Autodesk Fusion 360 part; units mm, degrees
note: some values were not read from the file. Set by a fixed rule: which sketch regions a step uses.
(part 3 of 3)
  arc A262 (-92.225, 45.1) -> (-92.725, 44.6) centre (-92.225, 44.6) ccw
  line L262 (-92.225, 45.1) -> (-79.225, 45.1)
  arc A263 (-78.725, 44.6) -> (-79.225, 45.1) centre (-79.225, 44.6) ccw
  line L263 (-78.725, 44.6) -> (-78.725, 31.6)
  arc A264 (-112.5625, 69.2) -> (-112.0625, 69.7) centre (-112.5625, 69.7) ccw
  line L264 (-112.5625, 69.2) -> (-125.5625, 69.2)
  arc A265 (-126.0625, 69.7) -> (-125.5625, 69.2) centre (-125.5625, 69.7) ccw
  line L265 (-126.0625, 69.7) -> (-126.0625, 82.7)
  arc A266 (-125.5625, 83.2) -> (-126.0625, 82.7) centre (-125.5625, 82.7) ccw
  line L266 (-125.5625, 83.2) -> (-112.5625, 83.2)
  arc A267 (-112.0625, 82.7) -> (-112.5625, 83.2) centre (-112.5625, 82.7) ccw
  line L267 (-112.0625, 82.7) -> (-112.0625, 69.7)
  arc A268 (-177.9688, 108.3) -> (-177.4687, 108.8) centre (-177.9688, 108.8) ccw
  line L268 (-177.9688, 108.3) -> (-183.9688, 108.3)
  arc A269 (-184.4688, 108.8) -> (-183.9688, 108.3) centre (-183.9688, 108.8) ccw
  line L269 (-184.4688, 108.8) -> (-184.4688, 122.8)
  arc A270 (-183.9688, 123.3) -> (-184.4687, 122.8) centre (-183.9687, 122.8) ccw
  line L270 (-183.9688, 123.3) -> (-177.9688, 123.3)
  arc A271 (-177.4688, 122.8) -> (-177.9688, 123.3) centre (-177.9688, 122.8) ccw
  line L271 (-177.4688, 122.8) -> (-177.4687, 108.8)
  arc A272 (-331.6375, 2.525) -> (-331.1375, 3.025) centre (-331.6375, 3.025) ccw
  line L272 (-331.6375, 2.525) -> (-344.6375, 2.525)
  arc A273 (-345.1375, 3.025) -> (-344.6375, 2.525) centre (-344.6375, 3.025) ccw
  line L273 (-345.1375, 3.025) -> (-345.1375, 16.025)
  arc A274 (-344.6375, 16.525) -> (-345.1375, 16.025) centre (-344.6375, 16.025) ccw
  line L274 (-344.6375, 16.525) -> (-331.6375, 16.525)
  arc A275 (-331.1375, 16.025) -> (-331.6375, 16.525) centre (-331.6375, 16.025) ccw
  line L275 (-331.1375, 16.025) -> (-331.1375, 3.025)
  arc A276 (-83.9875, 88.25) -> (-83.4875, 88.75) centre (-83.9875, 88.75) ccw
  line L276 (-83.9875, 88.25) -> (-96.9875, 88.25)
  arc A277 (-97.4875, 88.75) -> (-96.9875, 88.25) centre (-96.9875, 88.75) ccw
  line L277 (-97.4875, 88.75) -> (-97.4875, 101.75)
  arc A278 (-96.9875, 102.25) -> (-97.4875, 101.75) centre (-96.9875, 101.75) ccw
  line L278 (-96.9875, 102.25) -> (-83.9875, 102.25)
  arc A279 (-83.4875, 101.75) -> (-83.9875, 102.25) centre (-83.9875, 101.75) ccw
  line L279 (-83.4875, 101.75) -> (-83.4875, 88.75)
  arc A280 (-5.4063, 88.25) -> (-4.9063, 88.75) centre (-5.4062, 88.75) ccw
  line L280 (-5.4062, 88.25) -> (-18.4063, 88.25)
  arc A281 (-18.9062, 88.75) -> (-18.4063, 88.25) centre (-18.4062, 88.75) ccw
  line L281 (-18.9062, 88.75) -> (-18.9063, 101.75)
  arc A282 (-18.4062, 102.25) -> (-18.9063, 101.75) centre (-18.4063, 101.75) ccw
  line L282 (-18.4062, 102.25) -> (-5.4063, 102.25)
  arc A283 (-4.9062, 101.75) -> (-5.4063, 102.25) centre (-5.4062, 101.75) ccw
  line L283 (-4.9062, 101.75) -> (-4.9063, 88.75)
  arc A284 (-5.4063, 107.3) -> (-4.9062, 107.8) centre (-5.4063, 107.8) ccw
  line L284 (-5.4062, 107.3) -> (-18.4063, 107.3)
  arc A285 (-18.9062, 107.8) -> (-18.4063, 107.3) centre (-18.4062, 107.8) ccw
  line L285 (-18.9062, 107.8) -> (-18.9063, 120.8)
  arc A286 (-18.4062, 121.3) -> (-18.9063, 120.8) centre (-18.4062, 120.8) ccw
  line L286 (-18.4062, 121.3) -> (-5.4063, 121.3)
  arc A287 (-4.9062, 120.8) -> (-5.4063, 121.3) centre (-5.4063, 120.8) ccw
  line L287 (-4.9062, 120.8) -> (-4.9062, 107.8)
  arc A288 (-243.5313, 107.3) -> (-243.0313, 107.8) centre (-243.5312, 107.8) ccw
  line L288 (-243.5313, 107.3) -> (-256.5313, 107.3)
  arc A289 (-257.0312, 107.8) -> (-256.5312, 107.3) centre (-256.5312, 107.8) ccw
  line L289 (-257.0312, 107.8) -> (-257.0313, 120.8)
  arc A290 (-256.5312, 121.3) -> (-257.0312, 120.8) centre (-256.5312, 120.8) ccw
  line L290 (-256.5312, 121.3) -> (-243.5312, 121.3)
  arc A291 (-243.0313, 120.8) -> (-243.5313, 121.3) centre (-243.5313, 120.8) ccw
  line L291 (-243.0312, 120.8) -> (-243.0312, 107.8)
  arc A292 (-244.6183, 89.25) -> (-244.1182, 89.75) centre (-244.6183, 89.75) ccw
  line L292 (-244.6183, 89.25) -> (-250.6182, 89.25)
  arc A293 (-251.1182, 89.75) -> (-250.6182, 89.25) centre (-250.6182, 89.75) ccw
  line L293 (-251.1182, 89.75) -> (-251.1182, 103.75)
  arc A294 (-250.6182, 104.25) -> (-251.1182, 103.75) centre (-250.6182, 103.75) ccw
  line L294 (-250.6182, 104.25) -> (-244.6183, 104.25)
  arc A295 (-244.1183, 103.75) -> (-244.6183, 104.25) centre (-244.6182, 103.75) ccw
  line L295 (-244.1182, 103.75) -> (-244.1182, 89.75)
  arc A296 (-88.75, 50.15) -> (-88.25, 50.65) centre (-88.75, 50.65) ccw
  line L296 (-88.75, 50.15) -> (-101.75, 50.15)
  arc A297 (-102.25, 50.65) -> (-101.75, 50.15) centre (-101.75, 50.65) ccw
  line L297 (-102.25, 50.65) -> (-102.25, 63.65)
  arc A298 (-101.75, 64.15) -> (-102.25, 63.65) centre (-101.75, 63.65) ccw
  line L298 (-101.75, 64.15) -> (-88.75, 64.15)
  arc A299 (-88.25, 63.65) -> (-88.75, 64.15) centre (-88.75, 63.65) ccw
  line L299 (-88.25, 63.65) -> (-88.25, 50.65)
  arc A300 (-293.5375, 2.525) -> (-293.0375, 3.025) centre (-293.5375, 3.025) ccw
  line L300 (-293.5375, 2.525) -> (-306.5375, 2.525)
  arc A301 (-307.0375, 3.025) -> (-306.5375, 2.525) centre (-306.5375, 3.025) ccw
  line L301 (-307.0375, 3.025) -> (-307.0375, 16.025)
  arc A302 (-306.5375, 16.525) -> (-307.0375, 16.025) centre (-306.5375, 16.025) ccw
  line L302 (-306.5375, 16.525) -> (-293.5375, 16.525)
  arc A303 (-293.0375, 16.025) -> (-293.5375, 16.525) centre (-293.5375, 16.025) ccw
  line L303 (-293.0375, 16.025) -> (-293.0375, 3.025)
  arc A304 (-293.5375, 50.15) -> (-293.0375, 50.65) centre (-293.5375, 50.65) ccw
  line L304 (-293.5375, 50.15) -> (-306.5375, 50.15)
  arc A305 (-307.0375, 50.65) -> (-306.5375, 50.15) centre (-306.5375, 50.65) ccw
  line L305 (-307.0375, 50.65) -> (-307.0375, 63.65)
  arc A306 (-306.5375, 64.15) -> (-307.0375, 63.65) centre (-306.5375, 63.65) ccw
  line L306 (-306.5375, 64.15) -> (-293.5375, 64.15)
  arc A307 (-293.0375, 63.65) -> (-293.5375, 64.15) centre (-293.5375, 63.65) ccw
  line L307 (-293.0375, 63.65) -> (-293.0375, 50.65)
  arc A308 (-69.7, 50.15) -> (-69.2, 50.65) centre (-69.7, 50.65) ccw
  line L308 (-69.7, 50.15) -> (-82.7, 50.15)
  arc A309 (-83.2, 50.65) -> (-82.7, 50.15) centre (-82.7, 50.65) ccw
  line L309 (-83.2, 50.65) -> (-83.2, 63.65)
  arc A310 (-82.7, 64.15) -> (-83.2, 63.65) centre (-82.7, 63.65) ccw
  line L310 (-82.7, 64.15) -> (-69.7, 64.15)
  arc A311 (-69.2, 63.65) -> (-69.7, 64.15) centre (-69.7, 63.65) ccw
  line L311 (-69.2, 63.65) -> (-69.2, 50.65)
  arc A312 (-3.025, 31.1) -> (-2.525, 31.6) centre (-3.025, 31.6) ccw
  line L312 (-3.025, 31.1) -> (-16.025, 31.1)
  arc A313 (-16.525, 31.6) -> (-16.025, 31.1) centre (-16.025, 31.6) ccw
  line L313 (-16.525, 31.6) -> (-16.525, 44.6)
  arc A314 (-16.025, 45.1) -> (-16.525, 44.6) centre (-16.025, 44.6) ccw
  line L314 (-16.025, 45.1) -> (-3.025, 45.1)
  arc A315 (-2.525, 44.6) -> (-3.025, 45.1) centre (-3.025, 44.6) ccw
  line L315 (-2.525, 44.6) -> (-2.525, 31.6)
  arc A316 (-331.6375, 107.3) -> (-331.1375, 107.8) centre (-331.6375, 107.8) ccw
  line L316 (-331.6375, 107.3) -> (-344.6375, 107.3)
  arc A317 (-345.1375, 107.8) -> (-344.6375, 107.3) centre (-344.6375, 107.8) ccw
  line L317 (-345.1375, 107.8) -> (-345.1375, 120.8)
  arc A318 (-344.6375, 121.3) -> (-345.1375, 120.8) centre (-344.6375, 120.8) ccw
  line L318 (-344.6375, 121.3) -> (-331.6375, 121.3)
  arc A319 (-331.1375, 120.8) -> (-331.6375, 121.3) centre (-331.6375, 120.8) ccw
  line L319 (-331.1375, 120.8) -> (-331.1375, 107.8)
  arc A320 (-155.425, 31.1) -> (-154.925, 31.6) centre (-155.425, 31.6) ccw
  line L320 (-155.425, 31.1) -> (-168.425, 31.1)
  arc A321 (-168.925, 31.6) -> (-168.425, 31.1) centre (-168.425, 31.6) ccw
  line L321 (-168.925, 31.6) -> (-168.925, 44.6)
  arc A322 (-168.425, 45.1) -> (-168.925, 44.6) centre (-168.425, 44.6) ccw
  line L322 (-168.425, 45.1) -> (-155.425, 45.1)
  arc A323 (-154.925, 44.6) -> (-155.425, 45.1) centre (-155.425, 44.6) ccw
  line L323 (-154.925, 44.6) -> (-154.925, 31.6)
  arc A324 (-77.9688, 108.3) -> (-77.4687, 108.8) centre (-77.9688, 108.8) ccw
  line L324 (-77.9688, 108.3) -> (-83.9688, 108.3)
  arc A325 (-84.4688, 108.8) -> (-83.9688, 108.3) centre (-83.9687, 108.8) ccw
  line L325 (-84.4688, 108.8) -> (-84.4687, 122.8)
  arc A326 (-83.9688, 123.3) -> (-84.4687, 122.8) centre (-83.9688, 122.8) ccw
  line L326 (-83.9688, 123.3) -> (-77.9688, 123.3)
  arc A327 (-77.4688, 122.8) -> (-77.9688, 123.3) centre (-77.9688, 122.8) ccw
  line L327 (-77.4688, 122.8) -> (-77.4687, 108.8)
  arc A328 (-275.638, 32.1) -> (-275.138, 32.6) centre (-275.638, 32.6) ccw
  line L328 (-275.638, 32.1) -> (-281.638, 32.1)
  arc A329 (-282.138, 32.6) -> (-281.638, 32.1) centre (-281.638, 32.6) ccw
  line L329 (-282.138, 32.6) -> (-282.138, 46.6)
  arc A330 (-281.638, 47.1) -> (-282.138, 46.6) centre (-281.638, 46.6) ccw
  line L330 (-281.638, 47.1) -> (-275.638, 47.1)
  arc A331 (-275.138, 46.6) -> (-275.638, 47.1) centre (-275.638, 46.6) ccw
  line L331 (-275.138, 46.6) -> (-275.138, 32.6)
  arc A332 (-145.9, 50.15) -> (-145.4, 50.65) centre (-145.9, 50.65) ccw
  line L332 (-145.9, 50.15) -> (-158.9, 50.15)
  arc A333 (-159.4, 50.65) -> (-158.9, 50.15) centre (-158.9, 50.65) ccw
  line L333 (-159.4, 50.65) -> (-159.4, 63.65)
  arc A334 (-158.9, 64.15) -> (-159.4, 63.65) centre (-158.9, 63.65) ccw
  line L334 (-158.9, 64.15) -> (-145.9, 64.15)
  arc A335 (-145.4, 63.65) -> (-145.9, 64.15) centre (-145.9, 63.65) ccw
  line L335 (-145.4, 63.65) -> (-145.4, 50.65)
  arc A336 (-198.2875, 88.25) -> (-197.7875, 88.75) centre (-198.2875, 88.75) ccw
  line L336 (-198.2875, 88.25) -> (-211.2875, 88.25)
  arc A337 (-211.7875, 88.75) -> (-211.2875, 88.25) centre (-211.2875, 88.75) ccw
  line L337 (-211.7875, 88.75) -> (-211.7875, 101.75)
  arc A338 (-211.2875, 102.25) -> (-211.7875, 101.75) centre (-211.2875, 101.75) ccw
  line L338 (-211.2875, 102.25) -> (-198.2875, 102.25)
  arc A339 (-197.7875, 101.75) -> (-198.2875, 102.25) centre (-198.2875, 101.75) ccw
  line L339 (-197.7875, 101.75) -> (-197.7875, 88.75)
  arc A340 (-195.9063, 107.3) -> (-195.4063, 107.8) centre (-195.9063, 107.8) ccw
  line L340 (-195.9063, 107.3) -> (-208.9062, 107.3)
  arc A341 (-209.4062, 107.8) -> (-208.9062, 107.3) centre (-208.9062, 107.8) ccw
  line L341 (-209.4062, 107.8) -> (-209.4062, 120.8)
  arc A342 (-208.9062, 121.3) -> (-209.4063, 120.8) centre (-208.9062, 120.8) ccw
  line L342 (-208.9062, 121.3) -> (-195.9063, 121.3)
  arc A343 (-195.4063, 120.8) -> (-195.9063, 121.3) centre (-195.9063, 120.8) ccw
  line L343 (-195.4063, 120.8) -> (-195.4063, 107.8)
  arc A344 (-64.9375, 88.25) -> (-64.4375, 88.75) centre (-64.9375, 88.75) ccw
  line L344 (-64.9375, 88.25) -> (-77.9375, 88.25)
  arc A345 (-78.4375, 88.75) -> (-77.9375, 88.25) centre (-77.9375, 88.75) ccw
  line L345 (-78.4375, 88.75) -> (-78.4375, 101.75)
  arc A346 (-77.9375, 102.25) -> (-78.4375, 101.75) centre (-77.9375, 101.75) ccw
  line L346 (-77.9375, 102.25) -> (-64.9375, 102.25)
  arc A347 (-64.4375, 101.75) -> (-64.9375, 102.25) centre (-64.9375, 101.75) ccw
  line L347 (-64.4375, 101.75) -> (-64.4375, 88.75)
  arc A348 (-60.175, 2.525) -> (-59.675, 3.025) centre (-60.175, 3.025) ccw
  line L348 (-60.175, 2.525) -> (-73.175, 2.525)
  arc A349 (-73.675, 3.025) -> (-73.175, 2.525) centre (-73.175, 3.025) ccw
  line L349 (-73.675, 3.025) -> (-73.675, 16.025)
  arc A350 (-73.175, 16.525) -> (-73.675, 16.025) centre (-73.175, 16.025) ccw
  line L350 (-73.175, 16.525) -> (-60.175, 16.525)
  arc A351 (-59.675, 16.025) -> (-60.175, 16.525) centre (-60.175, 16.025) ccw
  line L351 (-59.675, 16.025) -> (-59.675, 3.025)
  arc A352 (-331.6375, 31.1) -> (-331.1375, 31.6) centre (-331.6375, 31.6) ccw
  line L352 (-331.6375, 31.1) -> (-344.6375, 31.1)
  arc A353 (-345.1375, 31.6) -> (-344.6375, 31.1) centre (-344.6375, 31.6) ccw
  line L353 (-345.1375, 31.6) -> (-345.1375, 44.6)
  arc A354 (-344.6375, 45.1) -> (-345.1375, 44.6) centre (-344.6375, 44.6) ccw
  line L354 (-344.6375, 45.1) -> (-331.6375, 45.1)
  arc A355 (-331.1375, 44.6) -> (-331.6375, 45.1) centre (-331.6375, 44.6) ccw
  line L355 (-331.1375, 44.6) -> (-331.1375, 31.6)
  arc A356 (-280.8438, 60.175) -> (-280.3438, 59.675) centre (-280.3438, 60.175) ccw
  line L356 (-280.8438, 60.175) -> (-280.8438, 73.175)
  arc A357 (-280.3438, 73.675) -> (-280.8438, 73.175) centre (-280.3438, 73.175) ccw
  line L357 (-280.3438, 73.675) -> (-267.3438, 73.675)
  arc A358 (-266.8438, 73.175) -> (-267.3438, 73.675) centre (-267.3438, 73.175) ccw
  line L358 (-266.8438, 73.175) -> (-266.8437, 60.175)
  arc A359 (-267.3438, 59.675) -> (-266.8438, 60.175) centre (-267.3438, 60.175) ccw
  line L359 (-267.3438, 59.675) -> (-280.3438, 59.675)
  arc A360 (-126.85, 2.525) -> (-126.35, 3.025) centre (-126.85, 3.025) ccw
  line L360 (-126.85, 2.525) -> (-139.85, 2.525)
  arc A361 (-140.35, 3.025) -> (-139.85, 2.525) centre (-139.85, 3.025) ccw
  line L361 (-140.35, 3.025) -> (-140.35, 16.025)
  arc A362 (-139.85, 16.525) -> (-140.35, 16.025) centre (-139.85, 16.025) ccw
  line L362 (-139.85, 16.525) -> (-126.85, 16.525)
  arc A363 (-126.35, 16.025) -> (-126.85, 16.525) centre (-126.85, 16.025) ccw
  line L363 (-126.35, 16.025) -> (-126.35, 3.025)
  arc A364 (-53.0313, 107.3) -> (-52.5312, 107.8) centre (-53.0313, 107.8) ccw
  line L364 (-53.0313, 107.3) -> (-66.0312, 107.3)
  arc A365 (-66.5312, 107.8) -> (-66.0312, 107.3) centre (-66.0312, 107.8) ccw
  line L365 (-66.5312, 107.8) -> (-66.5313, 120.8)
  arc A366 (-66.0313, 121.3) -> (-66.5313, 120.8) centre (-66.0312, 120.8) ccw
  line L366 (-66.0312, 121.3) -> (-53.0312, 121.3)
  arc A367 (-52.5313, 120.8) -> (-53.0313, 121.3) centre (-53.0312, 120.8) ccw
  line L367 (-52.5313, 120.8) -> (-52.5312, 107.8)
  arc A368 (-184, 50.15) -> (-183.5, 50.65) centre (-184, 50.65) ccw
  line L368 (-184, 50.15) -> (-197, 50.15)
  arc A369 (-197.5, 50.65) -> (-197, 50.15) centre (-197, 50.65) ccw
  line L369 (-197.5, 50.65) -> (-197.5, 63.65)
  arc A370 (-197, 64.15) -> (-197.5, 63.65) centre (-197, 63.65) ccw
  line L370 (-197, 64.15) -> (-184, 64.15)
  arc A371 (-183.5, 63.65) -> (-184, 64.15) centre (-184, 63.65) ccw
  line L371 (-183.5, 63.65) -> (-183.5, 50.65)
  arc A372 (-269.725, 2.525) -> (-269.225, 3.025) centre (-269.725, 3.025) ccw
  line L372 (-269.725, 2.525) -> (-282.725, 2.525)
  arc A373 (-283.225, 3.025) -> (-282.725, 2.525) centre (-282.725, 3.025) ccw
  line L373 (-283.225, 3.025) -> (-283.225, 16.025)
  arc A374 (-282.725, 16.525) -> (-283.225, 16.025) centre (-282.725, 16.025) ccw
  line L374 (-282.725, 16.525) -> (-269.725, 16.525)
  arc A375 (-269.225, 16.025) -> (-269.725, 16.525) centre (-269.725, 16.025) ccw
  line L375 (-269.225, 16.025) -> (-269.225, 3.025)
  arc A376 (-126.85, 50.15) -> (-126.35, 50.65) centre (-126.85, 50.65) ccw
  line L376 (-126.85, 50.15) -> (-139.85, 50.15)
  arc A377 (-140.35, 50.65) -> (-139.85, 50.15) centre (-139.85, 50.65) ccw
  line L377 (-140.35, 50.65) -> (-140.35, 63.65)
  arc A378 (-139.85, 64.15) -> (-140.35, 63.65) centre (-139.85, 63.65) ccw
  line L378 (-139.85, 64.15) -> (-126.85, 64.15)
  arc A379 (-126.35, 63.65) -> (-126.85, 64.15) centre (-126.85, 63.65) ccw
  line L379 (-126.35, 63.65) -> (-126.35, 50.65)
  arc A380 (-55.4125, 69.2) -> (-54.9125, 69.7) centre (-55.4125, 69.7) ccw
  line L380 (-55.4125, 69.2) -> (-68.4125, 69.2)
  arc A381 (-68.9125, 69.7) -> (-68.4125, 69.2) centre (-68.4125, 69.7) ccw
  line L381 (-68.9125, 69.7) -> (-68.9125, 82.7)
  arc A382 (-68.4125, 83.2) -> (-68.9125, 82.7) centre (-68.4125, 82.7) ccw
  line L382 (-68.4125, 83.2) -> (-55.4125, 83.2)
  arc A383 (-54.9125, 82.7) -> (-55.4125, 83.2) centre (-55.4125, 82.7) ccw
  line L383 (-54.9125, 82.7) -> (-54.9125, 69.7)
  arc A384 (-253.0563, 88.25) -> (-252.5563, 88.75) centre (-253.0563, 88.75) ccw
  line L384 (-253.0563, 88.25) -> (-266.0562, 88.25)
  arc A385 (-266.5562, 88.75) -> (-266.0563, 88.25) centre (-266.0563, 88.75) ccw
  line L385 (-266.5562, 88.75) -> (-266.5562, 101.75)
  arc A386 (-266.0562, 102.25) -> (-266.5562, 101.75) centre (-266.0563, 101.75) ccw
  line L386 (-266.0562, 102.25) -> (-253.0562, 102.25)
  arc A387 (-252.5562, 101.75) -> (-253.0562, 102.25) centre (-253.0562, 101.75) ccw
  line L387 (-252.5563, 101.75) -> (-252.5563, 88.75)
  arc A388 (-141.1375, 88.25) -> (-140.6375, 88.75) centre (-141.1375, 88.75) ccw
  line L388 (-141.1375, 88.25) -> (-154.1375, 88.25)
  arc A389 (-154.6375, 88.75) -> (-154.1375, 88.25) centre (-154.1375, 88.75) ccw
  line L389 (-154.6375, 88.75) -> (-154.6375, 101.75)
  arc A390 (-154.1375, 102.25) -> (-154.6375, 101.75) centre (-154.1375, 101.75) ccw
  line L390 (-154.1375, 102.25) -> (-141.1375, 102.25)
  arc A391 (-140.6375, 101.75) -> (-141.1375, 102.25) centre (-141.1375, 101.75) ccw
  line L391 (-140.6375, 101.75) -> (-140.6375, 88.75)
  arc A392 (-22.075, 31.1) -> (-21.575, 31.6) centre (-22.075, 31.6) ccw
  line L392 (-22.075, 31.1) -> (-35.075, 31.1)
  arc A393 (-35.575, 31.6) -> (-35.075, 31.1) centre (-35.075, 31.6) ccw
  line L393 (-35.575, 31.6) -> (-35.575, 44.6)
  arc A394 (-35.075, 45.1) -> (-35.575, 44.6) centre (-35.075, 44.6) ccw
  line L394 (-35.075, 45.1) -> (-22.075, 45.1)
  arc A395 (-21.575, 44.6) -> (-22.075, 45.1) centre (-22.075, 44.6) ccw
  line L395 (-21.575, 44.6) -> (-21.575, 31.6)
  arc A396 (-231.625, 2.525) -> (-231.125, 3.025) centre (-231.625, 3.025) ccw
  line L396 (-231.625, 2.525) -> (-244.625, 2.525)
  arc A397 (-245.125, 3.025) -> (-244.625, 2.525) centre (-244.625, 3.025) ccw
  line L397 (-245.125, 3.025) -> (-245.125, 16.025)
  arc A398 (-244.625, 16.525) -> (-245.125, 16.025) centre (-244.625, 16.025) ccw
  line L398 (-244.625, 16.525) -> (-231.625, 16.525)
  arc A399 (-231.125, 16.025) -> (-231.625, 16.525) centre (-231.625, 16.025) ccw
  line L399 (-231.125, 16.025) -> (-231.125, 3.025)
  arc A400 (-241.15, 50.15) -> (-240.65, 50.65) centre (-241.15, 50.65) ccw
  line L400 (-241.15, 50.15) -> (-254.15, 50.15)
  arc A401 (-254.65, 50.65) -> (-254.15, 50.15) centre (-254.15, 50.65) ccw
  line L401 (-254.65, 50.65) -> (-254.65, 63.65)
  arc A402 (-254.15, 64.15) -> (-254.65, 63.65) centre (-254.15, 63.65) ccw
  line L402 (-254.15, 64.15) -> (-241.15, 64.15)
  arc A403 (-240.65, 63.65) -> (-241.15, 64.15) centre (-241.15, 63.65) ccw
  line L403 (-240.65, 63.65) -> (-240.65, 50.65)
  arc A404 (-420.682, -4.942) -> (-410.182, -15.442) centre (-410.182, -4.942) ccw
  line L404 (-410.182, -15.442) -> (-409.932, -15.442)
  line L405 (-409.932, -15.442) -> (-409.932, -17.942)
  arc A405 (-409.932, -17.942) -> (-408.932, -18.942) centre (-408.932, -17.942) ccw
  line L406 (-408.932, -18.942) -> (-400.932, -18.942)
  arc A406 (-400.932, -18.942) -> (-399.932, -17.942) centre (-400.932, -17.942) ccw
  line L407 (-399.932, -17.942) -> (-399.932, -15.442)
  line L408 (-399.932, -15.442) -> (-358.7445, -15.442)
  line L409 (-358.7445, -15.442) -> (-358.7445, -17.942)
  arc A407 (-358.7445, -17.942) -> (-357.7445, -18.942) centre (-357.7445, -17.942) ccw
  line L410 (-357.7445, -18.942) -> (-349.7445, -18.942)
  arc A408 (-349.7445, -18.942) -> (-348.7445, -17.942) centre (-349.7445, -17.942) ccw
  line L411 (-348.7445, -17.942) -> (-348.7445, -15.442)
  line L412 (-348.7445, -15.442) -> (-307.557, -15.442)
  line L413 (-307.557, -15.442) -> (-307.557, -17.942)
  arc A409 (-307.557, -17.942) -> (-306.557, -18.942) centre (-306.557, -17.942) ccw
  line L414 (-306.557, -18.942) -> (-298.557, -18.942)
  arc A410 (-298.557, -18.942) -> (-297.557, -17.942) centre (-298.557, -17.942) ccw
  line L415 (-297.557, -17.942) -> (-297.557, -15.442)
  line L416 (-297.557, -15.442) -> (-256.3695, -15.442)
  line L417 (-256.3695, -15.442) -> (-256.3695, -17.942)
  arc A411 (-256.3695, -17.942) -> (-255.3695, -18.942) centre (-255.3695, -17.942) ccw
  line L418 (-255.3695, -18.942) -> (-247.3695, -18.942)
  arc A412 (-247.3695, -18.942) -> (-246.3695, -17.942) centre (-247.3695, -17.942) ccw
  line L419 (-246.3695, -17.942) -> (-246.3695, -15.442)
  line L420 (-246.3695, -15.442) -> (-205.182, -15.442)
  line L421 (-205.182, -15.442) -> (-205.182, -17.942)
  arc A413 (-205.182, -17.942) -> (-204.182, -18.942) centre (-204.182, -17.942) ccw
  line L422 (-204.182, -18.942) -> (-196.182, -18.942)
  arc A414 (-196.182, -18.942) -> (-195.182, -17.942) centre (-196.182, -17.942) ccw
  line L423 (-195.182, -17.942) -> (-195.182, -15.442)
  line L424 (-195.182, -15.442) -> (-153.9945, -15.442)
  line L425 (-153.9945, -15.442) -> (-153.9945, -17.942)
  arc A415 (-153.9945, -17.942) -> (-152.9945, -18.942) centre (-152.9945, -17.942) ccw
  line L426 (-152.9945, -18.942) -> (-144.9945, -18.942)
  arc A416 (-144.9945, -18.942) -> (-143.9945, -17.942) centre (-144.9945, -17.942) ccw
  line L427 (-143.9945, -17.942) -> (-143.9945, -15.442)
  line L428 (-143.9945, -15.442) -> (-102.807, -15.442)
  line L429 (-102.807, -15.442) -> (-102.807, -17.942)
  arc A417 (-102.807, -17.942) -> (-101.807, -18.942) centre (-101.807, -17.942) ccw
  line L430 (-101.807, -18.942) -> (-93.807, -18.942)
  arc A418 (-93.807, -18.942) -> (-92.807, -17.942) centre (-93.807, -17.942) ccw
  line L431 (-92.807, -17.942) -> (-92.807, -15.442)
  line L432 (-92.807, -15.442) -> (-51.6195, -15.442)
  line L433 (-51.6195, -15.442) -> (-51.6195, -17.942)
  arc A419 (-51.6195, -17.942) -> (-50.6195, -18.942) centre (-50.6195, -17.942) ccw
  line L434 (-50.6195, -18.942) -> (-42.6195, -18.942)
  arc A420 (-42.6195, -18.942) -> (-41.6195, -17.942) centre (-42.6195, -17.942) ccw
  line L435 (-41.6195, -17.942) -> (-41.6195, -15.442)
  line L436 (-41.6195, -15.442) -> (-0.432, -15.442)
  line L437 (-0.432, -15.442) -> (-0.432, -17.942)
  arc A421 (-0.432, -17.942) -> (0.568, -18.942) centre (0.568, -17.942) ccw
  line L438 (0.568, -18.942) -> (8.568, -18.942)
  arc A422 (8.568, -18.942) -> (9.568, -17.942) centre (8.568, -17.942) ccw
  line L439 (9.568, -17.942) -> (9.568, -15.442)
  line L440 (9.568, -15.442) -> (9.818, -15.442)
  arc A423 (9.818, -15.442) -> (20.318, -4.942) centre (9.818, -4.942) ccw
  line L441 (20.318, -4.942) -> (20.318, -4.692)
  line L442 (20.318, -4.692) -> (22.818, -4.692)
  arc A424 (22.818, -4.692) -> (23.818, -3.692) centre (22.818, -3.692) ccw
  line L443 (23.818, -3.692) -> (23.818, 4.308)
  arc A425 (23.818, 4.308) -> (22.818, 5.308) centre (22.818, 4.308) ccw
  line L444 (22.818, 5.308) -> (20.318, 5.308)
  line L445 (20.318, 5.308) -> (20.318, 25.183)
  line L446 (20.318, 25.183) -> (22.818, 25.183)
  arc A426 (22.818, 25.183) -> (23.818, 26.183) centre (22.818, 26.183) ccw
  line L447 (23.818, 26.183) -> (23.818, 34.183)
  arc A427 (23.818, 34.183) -> (22.818, 35.183) centre (22.818, 34.183) ccw
  line L448 (22.818, 35.183) -> (20.318, 35.183)
  line L449 (20.318, 35.183) -> (20.318, 55.058)
  line L450 (20.318, 55.058) -> (22.818, 55.058)
  arc A428 (22.818, 55.058) -> (23.818, 56.058) centre (22.818, 56.058) ccw
  line L451 (23.818, 56.058) -> (23.818, 64.058)
  arc A429 (23.818, 64.058) -> (22.818, 65.058) centre (22.818, 64.058) ccw
  line L452 (22.818, 65.058) -> (20.318, 65.058)
  line L453 (20.318, 65.058) -> (20.318, 84.933)
  line L454 (20.318, 84.933) -> (22.818, 84.933)
  arc A430 (22.818, 84.933) -> (23.818, 85.933) centre (22.818, 85.933) ccw
  line L455 (23.818, 85.933) -> (23.818, 93.933)
  arc A431 (23.818, 93.933) -> (22.818, 94.933) centre (22.818, 93.933) ccw
  line L456 (22.818, 94.933) -> (20.318, 94.933)
  line L457 (20.318, 94.933) -> (20.318, 114.808)
  line L458 (20.318, 114.808) -> (22.818, 114.808)
  arc A432 (22.818, 114.808) -> (23.818, 115.808) centre (22.818, 115.808) ccw
  line L459 (23.818, 115.808) -> (23.818, 123.808)
  arc A433 (23.818, 123.808) -> (22.818, 124.808) centre (22.818, 123.808) ccw
  line L460 (22.818, 124.808) -> (20.318, 124.808)
  line L461 (20.318, 124.808) -> (20.318, 125.058)
  arc A434 (20.318, 125.058) -> (9.818, 135.558) centre (9.818, 125.058) ccw
  line L462 (9.818, 135.558) -> (9.568, 135.558)
  line L463 (9.568, 135.558) -> (9.568, 138.058)
  arc A435 (9.568, 138.058) -> (8.568, 139.058) centre (8.568, 138.058) ccw
  line L464 (8.568, 139.058) -> (0.568, 139.058)
  arc A436 (0.568, 139.058) -> (-0.432, 138.058) centre (0.568, 138.058) ccw
  line L465 (-0.432, 138.058) -> (-0.432, 135.558)
  line L466 (-0.432, 135.558) -> (-41.6195, 135.558)
  line L467 (-41.6195, 135.558) -> (-41.6195, 138.058)
  arc A437 (-41.6195, 138.058) -> (-42.6195, 139.058) centre (-42.6195, 138.058) ccw
  line L468 (-42.6195, 139.058) -> (-50.6195, 139.058)
  arc A438 (-50.6195, 139.058) -> (-51.6195, 138.058) centre (-50.6195, 138.058) ccw
  line L469 (-51.6195, 138.058) -> (-51.6195, 135.558)
  line L470 (-51.6195, 135.558) -> (-92.807, 135.558)
  line L471 (-92.807, 135.558) -> (-92.807, 138.058)
  arc A439 (-92.807, 138.058) -> (-93.807, 139.058) centre (-93.807, 138.058) ccw
  line L472 (-93.807, 139.058) -> (-101.807, 139.058)
  arc A440 (-101.807, 139.058) -> (-102.807, 138.058) centre (-101.807, 138.058) ccw
  line L473 (-102.807, 138.058) -> (-102.807, 135.558)
  line L474 (-102.807, 135.558) -> (-143.9945, 135.558)
  line L475 (-143.9945, 135.558) -> (-143.9945, 138.058)
  arc A441 (-143.9945, 138.058) -> (-144.9945, 139.058) centre (-144.9945, 138.058) ccw
  line L476 (-144.9945, 139.058) -> (-152.9945, 139.058)
  arc A442 (-152.9945, 139.058) -> (-153.9945, 138.058) centre (-152.9945, 138.058) ccw
  line L477 (-153.9945, 138.058) -> (-153.9945, 135.558)
  line L478 (-153.9945, 135.558) -> (-195.182, 135.558)
  line L479 (-195.182, 135.558) -> (-195.182, 138.058)
  arc A443 (-195.182, 138.058) -> (-196.182, 139.058) centre (-196.182, 138.058) ccw
  line L480 (-196.182, 139.058) -> (-204.182, 139.058)
  arc A444 (-204.182, 139.058) -> (-205.182, 138.058) centre (-204.182, 138.058) ccw
  line L481 (-205.182, 138.058) -> (-205.182, 135.558)
  line L482 (-205.182, 135.558) -> (-246.3695, 135.558)
  line L483 (-246.3695, 135.558) -> (-246.3695, 138.058)
  arc A445 (-246.3695, 138.058) -> (-247.3695, 139.058) centre (-247.3695, 138.058) ccw
  line L484 (-247.3695, 139.058) -> (-255.3695, 139.058)
  arc A446 (-255.3695, 139.058) -> (-256.3695, 138.058) centre (-255.3695, 138.058) ccw
  line L485 (-256.3695, 138.058) -> (-256.3695, 135.558)
  line L486 (-256.3695, 135.558) -> (-297.557, 135.558)
  line L487 (-297.557, 135.558) -> (-297.557, 138.058)
  arc A447 (-297.557, 138.058) -> (-298.557, 139.058) centre (-298.557, 138.058) ccw
  line L488 (-298.557, 139.058) -> (-306.557, 139.058)
  arc A448 (-306.557, 139.058) -> (-307.557, 138.058) centre (-306.557, 138.058) ccw
  line L489 (-307.557, 138.058) -> (-307.557, 135.558)
  line L490 (-307.557, 135.558) -> (-348.7445, 135.558)
  line L491 (-348.7445, 135.558) -> (-348.7445, 138.058)
  arc A449 (-348.7445, 138.058) -> (-349.7445, 139.058) centre (-349.7445, 138.058) ccw
  line L492 (-349.7445, 139.058) -> (-357.7445, 139.058)
  arc A450 (-357.7445, 139.058) -> (-358.7445, 138.058) centre (-357.7445, 138.058) ccw
  line L493 (-358.7445, 138.058) -> (-358.7445, 135.558)
  line L494 (-358.7445, 135.558) -> (-399.932, 135.558)
  line L495 (-399.932, 135.558) -> (-399.932, 138.058)
  arc A451 (-399.932, 138.058) -> (-400.932, 139.058) centre (-400.932, 138.058) ccw
  line L496 (-400.932, 139.058) -> (-408.932, 139.058)
  arc A452 (-408.932, 139.058) -> (-409.932, 138.058) centre (-408.932, 138.058) ccw
  line L497 (-409.932, 138.058) -> (-409.932, 135.558)
  line L498 (-409.932, 135.558) -> (-410.182, 135.558)
  arc A453 (-410.182, 135.558) -> (-420.682, 125.058) centre (-410.182, 125.058) ccw
  line L499 (-420.682, 125.058) -> (-420.682, 94.933)
  line L500 (-420.682, 94.933) -> (-423.182, 94.933)
  arc A454 (-423.182, 94.933) -> (-424.182, 93.933) centre (-423.182, 93.933) ccw
  line L501 (-424.182, 93.933) -> (-424.182, 85.933)
  arc A455 (-424.182, 85.933) -> (-423.182, 84.933) centre (-423.182, 85.933) ccw
  line L502 (-423.182, 84.933) -> (-420.682, 84.933)
  line L503 (-420.682, 84.933) -> (-420.682, 65.058)
  line L504 (-420.682, 65.058) -> (-423.182, 65.058)
  arc A456 (-423.182, 65.058) -> (-424.182, 64.058) centre (-423.182, 64.058) ccw
  line L505 (-424.182, 64.058) -> (-424.182, 56.058)
  arc A457 (-424.182, 56.058) -> (-423.182, 55.058) centre (-423.182, 56.058) ccw
  line L506 (-423.182, 55.058) -> (-420.682, 55.058)
  line L507 (-420.682, 55.058) -> (-420.682, 5.308)
  line L508 (-420.682, 5.308) -> (-423.182, 5.308)
  arc A458 (-423.182, 5.308) -> (-424.182, 4.308) centre (-423.182, 4.308) ccw
  line L509 (-424.182, 4.308) -> (-424.182, -3.692)
  arc A459 (-424.182, -3.692) -> (-423.182, -4.692) centre (-423.182, -3.692) ccw
  line L510 (-423.182, -4.692) -> (-420.682, -4.692)
  line L511 (-420.682, -4.692) -> (-420.682, -4.942)
  line L512 (-371.82, 33.914) -> (-402.52, 33.914)
  line L513 (-402.52, 33.914) -> (-402.52, 65.774)
  line L514 (-402.52, 65.774) -> (-371.82, 65.774)
  line L515 (-371.82, 65.774) -> (-371.82, 33.914)
  line L516 (-396.17, 44.414) -> (-378.17, 44.414)
  line L517 (-374.67, 40.914) -> (-374.67, 32.914)
  line L518 (-378.17, 29.414) -> (-396.17, 29.414)
  line L519 (-399.67, 32.914) -> (-399.67, 40.914)
  line L520 (-399.67, 44.414) -> (-374.67, 29.414) construction
  line L521 (-374.67, 44.414) -> (-399.67, 29.414) construction
  arc A460 (-378.17, 29.414) -> (-374.67, 32.914) centre (-378.17, 32.914) ccw
  arc A461 (-374.67, 40.914) -> (-378.17, 44.414) centre (-378.17, 40.914) ccw
  arc A462 (-396.17, 44.414) -> (-399.67, 40.914) centre (-396.17, 40.914) ccw
  arc A463 (-399.67, 32.914) -> (-396.17, 29.414) centre (-396.17, 32.914) ccw
  point P0 (-387.17, 36.914)
  dimension "d88" = 18.162
  dimension "d89" = 49.356
  dimension "d90" = 31.86
  dimension "d91" = 30.7
  dimension "d92" = 25
  dimension "d93" = 15
  dimension "d94" = 3.5
  dimension "d95" = 15.35
  dimension "d96" = 3
  constraint horizontal L512
  constraint vertical L513
  constraint horizontal L514
  constraint vertical L515
  constraint horizontal L516
  constraint perpendicular L516 L517
  constraint parallel L516 L518
  constraint parallel L517 L519
  constraint coincident L520 P0
  constraint coincident L521 P0
  constraint coincident L520.end L517
  constraint coincident L520.end L518
  constraint tangent L517 A460
  constraint tangent L518 A460
  constraint coincident L521.start L517
  constraint coincident L521.start L516
  constraint tangent L517 A461
  constraint tangent L516 A461
  constraint equal A460 A461
  constraint coincident L520.start L516
  constraint coincident L520.start L519
  constraint tangent L516 A462
  constraint tangent L519 A462
  constraint equal A460 A462
  constraint coincident L521.end L519
  constraint coincident L521.end L518
  constraint tangent L519 A463
  constraint tangent L518 A463
  constraint equal A460 A463
  measures "d88" distance of L507 L513
  measures "d89" distance of L408 L512
  measures "d90" distance of L512 L514
  measures "d91" distance of L513 L515
  measures "d92" distance of L520.end L521.end
  measures "d93" distance of L521.start L520.end
  measures "d94" radius of A460
  measures "d95" distance of L515 P0
  measures "d96" distance of L512 P0
extrude "Extrude9" cut sketch "Sketch3" against normal blind 10 contours L512 L517 L518 L519 A460 A463 | L512 L516 L517 L519 A461 A462
equation "d88 = 18.662 mm - 0.5 mm"
equation "d89 = 49.856 mm - 0.5 mm"
equation "d95 = ( 30.70 / 2 ) * 1 mm"
